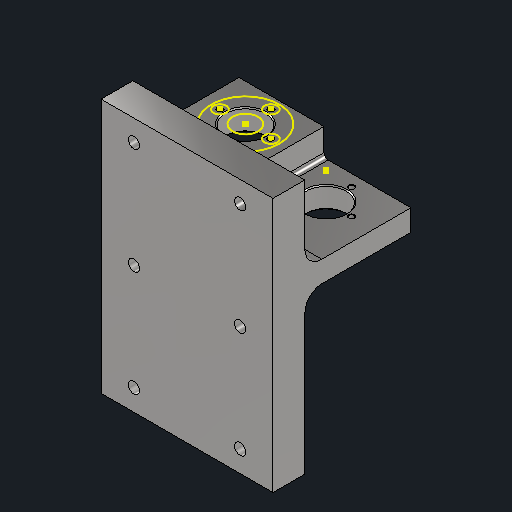
# Autodesk Inventor part: KN-00-02-05
Saved by Autodesk Inventor 2025.2 (Build 292293000, 293)
## iProperties
Created: 2025-04-13
Part Number: KN-00-02-05
Material: X5CrNi18-10
Document SubType Name: Modeling
Designer: Kacper Mik
Density: 8 g/cm^3
Appearance: Semi-Polished
Mass: 1464.75 g
Surface Area: 369.846 cm^2
Volume: 183.094 cm^3
Author: Kacper Mik
Autodesk Inventor part; units mm, degrees
ref_plane "YZ Plane" through (0, 0, 0) normal (1, 0, 0) x (0, 1, 0)
ref_plane "XZ Plane" through (0, 0, 0) normal (0, 1, 0) x (-1, 0, 0)
ref_plane "XY Plane" through (0, 0, 0) normal (0, 0, 1) x (1, 0, 0)
sketch "Sketch1" plane through (0, 0, 0) normal (0, 1, 0) x (-1, 0, 0)
  line L0 (-22.5, 17.5) -> (22.5, 17.5)
  line L1 (22.5, 17.5) -> (22.5, -17.5)
  line L2 (22.5, -17.5) -> (-22.5, -17.5)
  line L3 (-22.5, -17.5) -> (-22.5, 17.5)
  line L4 (-22.5, 17.5) -> (22.5, -17.5) construction
  line L5 (22.5, 17.5) -> (-22.5, -17.5) construction
  point P0 (0, 0)
  dimension "d0" = 45
  dimension "d1" = 35
  constraints: 12 end point, 2 midpoint, 2 parallel, 1 horizontal, 1 perpendicular
  measures "d0" distance of L1.end L2.end
  measures "d1" distance of L0.end L1.end
extrude "Extrusion1" add sketch "Sketch1" along normal mid plane 10
sketch "Sketch2" plane through (0, 5, 0) normal (0, 1, 0) x (1, 0, 0)
  point P0 (0, 0)
  point P1 (0, 0)
  constraints: 1 coincident
hole "Hole1" at (0, 5, 0) direction (0, -1, 0) diameter 19 end through all
sketch "Sketch3" plane through (0, 5, 0) normal (0, 1, 0) x (1, 0, 0)
  circle A0 centre (0, 0) radius 12 construction
  point P0 (0, 12)
  point P1 (12, 0)
  point P2 (0, -12)
  point P3 (-12, 0)
  dimension "d11" = 24
  constraints: 4 point on circle, 2 horizontal alignment, 2 vertical alignment, 1 centre point, 1 coincident
  measures "d11" diameter of A0
hole "Hole2" at (0, 5, -12) at (12, 5, 0) at (0, 5, 12) at (-12, 5, 0) direction (0, -1, 0) diameter 2.459 end through all thread size "M3x0.5" class "6H" standard "ISO Metric profile"
chamfer "Chamfer1" distance 0.2 angle 45 4 edges at (0, 5, -13.2295) (12, 5, -1.2295) (-12, 5, -1.2295) (0, 5, 10.7705)
chamfer "Chamfer2" distance 0.5 angle 45 2 edges at (0, 5, -9.5) (0, -5, -9.5)
sketch "Sketch4" plane through (-22.5, -5, 17.5) normal (0, 0, 1) x (1, 0, 0)
  line L0 (45, 0) -> (0, 0) projected
  line L1 (45, 0) -> (45, 10) projected
  line L2 (0, 10) -> (45, 10) projected
  line L3 (0, 0) -> (0, 10) projected
  point P0 (22.5, 5)
extrude "1" add sketch "Sketch4" along normal blind 15
sketch "Sketch7" plane through (-22.5, -5, 32.5) normal (0, 0, 1) x (1, 0, 0)
  line L0 (45, 10) -> (0, 10) construction
  line L1 (0, 10) -> (0, 0) construction
  line L2 (0, 0) -> (45, 0) construction
  line L3 (45, 0) -> (45, 10) construction
  line L4 (4, 10) -> (4, 22.65)
  line L5 (0, 10) -> (4, 10)
  line L6 (4, 22.65) -> (-36, 22.65)
  line L7 (6.5, 15) -> (6.5, 10) construction
  line L8 (0.5, 27.65) -> (0.5, 22.65) construction
  line L9 (-36, 12.65) -> (-36, 22.65)
  line L10 (-36, 12.65) -> (0, 12.65)
  line L11 (0, 12.65) -> (0, 10)
  point P0 (22.5, 5)
  dimension "d46" = 12.65
  dimension "d47" = 45
  dimension "d49" = 40
  dimension "d75" = 10
  constraints: 16 end point, 2 horizontal, 2 vertical, 1 collinear, 1 perpendicular, 1 point on line, 4 other
  measures "d46" distance of L4.start L4.end
  measures "d47" distance of L1.end L2.end
  measures "d49" distance of L4.end L6.end
  measures "d75" distance of L9.start L6.end
extrude "2" add sketch "Sketch7" against normal up to surface (50 mm away)
sketch "Sketch8" plane through (-58.5, 17.65, 32.5) normal (0, 1, 0) x (1, 0, 0)
  circle A0 centre (20.5, 32.5) radius 16 projected
  circle A1 centre (32.5, 32.5) radius 3 projected
  circle A2 centre (20.5, 20.5) radius 3 projected
  circle A3 centre (8.5, 32.5) radius 3 projected
  circle A4 centre (20.5, 44.5) radius 3 projected
  circle A5 centre (20.5, 32.5) radius 6 projected
  point P0 (58.5, 32.5)
hole "Hole4" at (-38, 17.65, 0) direction (0, -1, 0) diameter 19 end through all
hole "Hole5" at (-38, 17.65, -12) at (-26, 17.65, 0) at (-38, 17.65, 12) at (-50, 17.65, 0) direction (0, -1, 0) diameter 2.459 end through all thread size "M3x0.5" class "6H" standard "ISO Metric profile"
chamfer "Chamfer4" distance 0.2 angle 45 4 edges at (-38, 17.65, -13.2295) (-26, 17.65, -1.2295) (-50, 17.65, -1.2295) (-38, 17.65, 10.7705)
chamfer "Chamfer5" distance 0.5 angle 45 2 edges at (-38, 17.65, -9.5) (-38, 7.65, -9.5)
sketch "Sketch9" plane through (-22.5, -5, 32.5) normal (0, 0, 1) x (1, 0, 0)
  line L0 (-36, 22.65) -> (-36, 12.65) construction
  line L1 (0, 0) -> (45, 0) construction
  line L2 (-36, 22.65) -> (45, 22.65) construction
  line L3 (45, 22.65) -> (45, 0) construction
  line L4 (45, 0) -> (-36, 0) construction
  line L5 (-36, 0) -> (-36, 22.65) construction
  line L6 (-36, 22.65) -> (45, 0) construction
  line L7 (45, 22.65) -> (-36, 0) construction
  line L8 (45, -23.675) -> (-36, -23.675)
  line L9 (-36, -23.675) -> (-36, 46.325)
  line L10 (-36, 46.325) -> (45, 46.325)
  line L11 (45, 46.325) -> (45, -23.675)
  line L12 (45, -23.675) -> (-36, 46.325) construction
  line L13 (-36, -23.675) -> (45, 46.325) construction
  point P0 (22.5, 5)
  point P1 (4.5, 11.325)
  dimension "d76" = 81
  dimension "d77" = 70
  constraints: 24 end point, 4 parallel, 3 midpoint, 2 horizontal, 2 perpendicular
  measures "d76" distance of L9.end L10.end
  measures "d77" distance of L8.end L9.end
extrude "Extrusion5" add sketch "Sketch9" along normal blind 15
sketch "Sketch11" plane through (-58.5, -28.675, 32.5) normal (0, -1, 0) x (1, 0, 0)
  line L0 (0, 0) -> (81, 0) projected
  line L1 (81, 0) -> (81, 15) projected
  line L2 (0, 15) -> (81, 15) projected
  line L3 (0, 0) -> (0, 15) projected
  point P0 (58.5, -32.5)
extrude "Extrusion6" add sketch "Sketch11" along normal blind 50
sketch "Sketch10" plane through (-22.5, -5, 47.5) normal (0, 0, 1) x (1, 0, 0)
  line L0 (45, 46.325) -> (-36, 46.325) construction
  line L1 (-36, 46.325) -> (-36, -73.675) construction
  line L2 (45, 46.325) -> (45, -73.675) construction
  line L3 (-36, 46.325) -> (-36, -23.675) construction
  line L4 (-20.5, -13.675) -> (29.5, -13.675) construction
  line L5 (29.5, -13.675) -> (29.5, 36.325) construction
  line L6 (29.5, 36.325) -> (-20.5, 36.325) construction
  line L7 (-20.5, 36.325) -> (-20.5, -13.675) construction
  line L8 (-20.5, -13.675) -> (29.5, 36.325) construction
  line L9 (29.5, -13.675) -> (-20.5, 36.325) construction
  line L10 (45, -73.675) -> (-36, -73.675) projected
  point P0 (4.5, 11.325)
  point P1 (-20.5, -63.675)
  point P2 (29.5, -63.675)
  dimension "d80" = 50
  dimension "d81" = 50
  dimension "d91" = 40.5
  dimension "d92" = 35
  dimension "d93" = 50
  constraints: 12 end point, 4 coincident, 2 midpoint, 2 parallel, 2 vertical alignment, 1 horizontal, 1 horizontal alignment, 1 perpendicular
  measures "d80" distance of L6.end L5.end
  measures "d81" distance of L5.end L4.end
  measures "d91" distance from line of L2 point (4.5, 11.325)
  measures "d92" distance from line of L0 point (4.5, 11.325)
  measures "d93" distance of point (29.5, -63.675) point (29.5, -13.675)
hole "Hole6" at (-43, 31.325, 47.5) at (7, 31.325, 47.5) at (7, -18.675, 47.5) at (-43, -18.675, 47.5) at (7, -68.675, 47.5) at (-43, -68.675, 47.5) direction (0, 0, -1) diameter 5.3 end through all clearance for "Hex Head Cap Screw ISO 24017" size "M5" standard "ISO"
fillet "Fillet2" radius 8 4 edges at (0, -5, 32.5) (-40.5, 7.65, 32.5) (-38.5, 17.65, 32.5) (2, 5, 32.5)
fillet "Fillet3" radius 2 4 edges at (-18.5, 7.3431, 30.1569) (-18.5, 15.325, 32.5) (-18.5, 5, 3.5) (-22.5, 7.65, 3.5)
chamfer "Chamfer6" distance 0.2 angle 45 4 edges at (-43, -16.025, 32.5) (7, -16.025, 32.5) (-43, 33.975, 32.5) (7, 33.975, 32.5)
body "Solid1"
